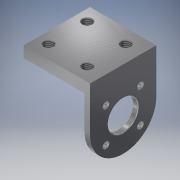
# Autodesk Inventor part: Winkelhaak
Saved by Autodesk Inventor 2018 (Build 220112000, 112)
## iProperties
Created: 2018-02-20
Part Number: Winkelhaak
Material: Steel
Document SubType Name: Modeling
Designer: ruben
Density: 7.85 g/cm^3
Sheet Metal Rule: Default_mm
Appearance: Machined - Aluminum
Mass: 381.572 g
Surface Area: 171.104 cm^2
Volume: 48.6079 cm^3
Author: ruben
Autodesk Inventor part; units mm, degrees
ref_plane "YZ Plane" through (0, 0, 0) normal (1, 0, 0) x (0, 1, 0)
ref_plane "XZ Plane" through (0, 0, 0) normal (0, 1, 0) x (-1, 0, 0)
ref_plane "XY Plane" through (0, 0, 0) normal (0, 0, 1) x (1, 0, 0)
sketch "Sketch3" plane through (0, 0, 0) normal (0, 0, 1) x (1, 0, 0)
  line L0 (0, -70) -> (0, 0)
  line L1 (0, 0) -> (-60, 0)
  line L2 (-60, 0) -> (-60, -10)
  line L3 (-60, -10) -> (-5, -10)
  line L4 (-5, -10) -> (-5, -70)
  line L5 (-5, -70) -> (0, -70)
  dimension "d0" = 5
  dimension "d1" = 10
  dimension "d2" = 70
  dimension "d3" = 60
  constraints: 12 end point, 3 perpendicular, 2 vertical, 1 horizontal
  measures "d0" distance between parallel lines of L4 L0
  measures "d1" distance between parallel lines of L1 L3
  measures "d2" distance between parallel lines of L1 L5
  measures "d3" distance between parallel lines of L2 L0
extrude "Extrusion1" add sketch "Sketch3" along normal mid plane 60
sketch "Sketch4" plane through (-60, -10, 30) normal (0, -1, 0) x (1, 0, 0)
  line L0 (10, -12.5) -> (45, -12.5)
  line L1 (45, -12.5) -> (45, -47.5)
  line L2 (45, -47.5) -> (10, -47.5)
  line L3 (10, -47.5) -> (10, -12.5)
  line L4 (10, -12.5) -> (45, -47.5) construction
  line L5 (45, -12.5) -> (10, -47.5) construction
  line L6 (55, -60) -> (0, -60) projected
  line L7 (0, 0) -> (55, 0) projected
  line L8 (0, 0) -> (0, -60) projected
  line L9 (55, 0) -> (55, -60) projected
  point P0 (60, -30)
  point P1 (27.5, -30)
  dimension "d6" = 35
  dimension "d7" = 35
  dimension "d8" = 30
  dimension "d9" = 60
  dimension "d10" = 27.5
  dimension "d11" = 55
  constraints: 12 end point, 4 coincident, 2 midpoint, 2 parallel, 1 horizontal, 1 perpendicular
  measures "d6" distance of L1.end L2.end
  measures "d7" distance of L0.end L1.end
  measures "d8" distance from line of L6 point (27.5, -30)
  measures "d9" distance between parallel lines of L6 L7
  measures "d10" distance from line of L8 point (27.5, -30)
  measures "d11" distance between parallel lines of L8 L9
hole "Hole1" at (-15, -10, 17.5) at (-15, -10, -17.5) at (-50, -10, -17.5) at (-50, -10, 17.5) direction (0, 1, 0) diameter 8.376 end through all thread size "M10x1.5" class "6H" standard "ISO Metric profile"
sketch "Sketch5" plane through (0, -70, 30) normal (1, 0, 0) x (0, 0, -1)
  line L0 (347.401, -568.181) -> (340.7975, -584.7897)
  line L1 (-15.5128, -15.5128) -> (63.4595, 63.4595) construction
  line L2 (77.4824, -17.4824) -> (-3.7678, 63.7678) construction
  circle A0 centre (30, 30) radius 22 construction
  line L3 (60, 70) -> (0, 70) projected
  line L4 (0, 0) -> (0, 70) projected
  line L5 (60, 70) -> (60, 0) projected
  point P0 (14.4437, 45.5563)
  point P1 (14.4437, 14.4437)
  point P2 (45.5563, 14.4437)
  point P3 (45.5563, 45.5563)
  point P4 (0, 60)
  point P5 (60, 60)
  dimension "d49" = 44
  constraints: 10 point on line, 6 end point, 4 point on circle, 1 centre point, 1 coincident
  measures "d49" diameter of A0
fillet "Fillet1" radius 30 2 edges at (-2.5, -70, -30) (-2.5, -70, 30)
hole "Hole5" at (0, -24.4437, 15.5563) at (0, -24.4437, -15.5563) at (0, -55.5563, -15.5563) at (0, -55.5563, 15.5563) direction (-1, 0, 0) diameter 4 end through all countersink diameter 6 countersink angle 90
hole "Hole6" at (0, -40, 0) direction (-1, 0, 0) diameter 27 depth 8
chamfer "Chamfer1" distance 0.5 angle 45 6 edges at (0, -40, 13.5) (-5, -40, 13.5) (-5, -24.4437, 17.5563) (-5, -24.4437, -13.5563) (-5, -55.5563, -13.5563) (-5, -55.5563, 17.5563)
chamfer "Chamfer2" distance 0.5 angle 45 8 edges at (-15, 0, 21.688) (-15, 0, -13.312) (-50, 0, -13.312) (-50, 0, 21.688) (-15, -10, 21.688) (-15, -10, -13.312) (-50, -10, 21.688) (-50, -10, -13.312)
equation "\"d8\" = 0.5 * d9"
equation "\"d10\" = 0.5 * d11"
equation "\"BendRadius\" = Thickness"
equation "\"BendReliefWidth\" = Thickness"
equation "\"BendReliefDepth\" = 0.5 * Thickness"
equation "\"CornerReliefSize\" = 4 * Thickness"
equation "\"MinimumRemnant\" = 2 * Thickness"
equation "\"TransitionRadius\" = BendRadius"
equation "\"JacobiRadiusSize\" = BendRadius"
equation "\"GapSize\" = Thickness"
equation "\"Thickness\" = 0.5"
body "Solid1"
